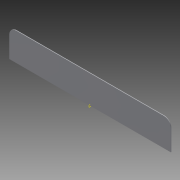
# Autodesk Inventor part: FE00036Shelf
Saved by Autodesk Inventor 2013 (Build 170138000, 138)
## iProperties
Created: 2013-01-14
Part Number: FE00036Shelf
Material: Aluminum 6061
Document SubType Name: Modeling
Designer: Phillip
Density: 1 g/cm^3
d0: 69.000 in
d1: 12.000 in
d2: 0.250 in
d3: 0.00 deg
d4: 3.000 in
Author: Phillip
Autodesk Inventor part; units mm, degrees
ref_plane "YZ Plane" through (0, 0, 0) normal (1, 0, 0) x (0, 1, 0)
ref_plane "XZ Plane" through (0, 0, 0) normal (0, 1, 0) x (-1, 0, 0)
ref_plane "XY Plane" through (0, 0, 0) normal (0, 0, 1) x (1, 0, 0)
sketch "Sketch1" plane through (0, 0, 0) normal (0, 0, 1) x (1, 0, 0)
  line L0 (0, 0) -> (1752.6, 0)
  line L1 (1752.6, 0) -> (1752.6, 304.8)
  line L2 (1752.6, 304.8) -> (0, 304.8)
  line L3 (0, 304.8) -> (0, 0)
  dimension "d0" = 1752.6
  dimension "d1" = 304.8
  constraints: 8 end point, 2 parallel, 1 horizontal, 1 perpendicular
  measures "d0" distance of L2.end L1.end
  measures "d1" distance of L1.end L0.end
extrude "Extrusion1" add sketch "Sketch1" against normal blind 6.35
fillet "Fillet1" radius 76.2 2 edges at (0, 304.8, -3.175) (1752.6, 304.8, -3.175)
ref_plane "Work Plane1" through (876.3, 0, 0) normal (1, 0, 0) x (0, 1, 0)
body "Solid1"
